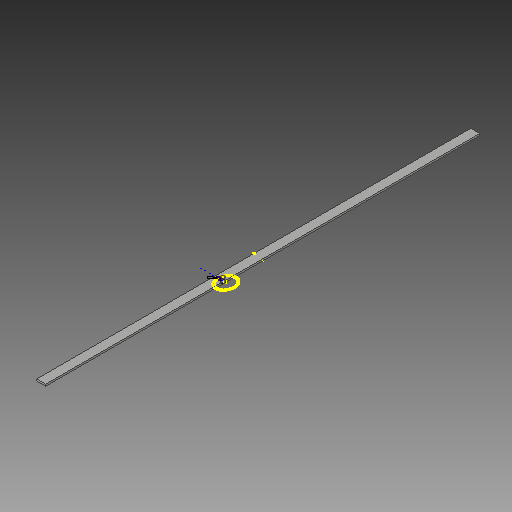
# Autodesk Inventor part: håndfang
Saved by Autodesk Inventor 2018 (Build 220112000, 112)
## iProperties
Created: 2019-09-28
Part Number: håndfang
Material: S235JR
Document SubType Name: Modeling
Designer: loppen
Density: 7.85 g/cm^3
Appearance: Light Gray
Mass: 1186.28 g
Surface Area: 727.87 cm^2
Volume: 151.119 cm^3
Author: loppen
Autodesk Inventor part; units mm, degrees
ref_plane "YZ Plane" through (0, 0, 0) normal (1, 0, 0) x (0, 1, 0)
ref_plane "XZ Plane" through (0, 0, 0) normal (0, 1, 0) x (-1, 0, 0)
ref_plane "XY Plane" through (0, 0, 0) normal (0, 0, 1) x (1, 0, 0)
sketch "Sketch1" plane through (0, 0, 0) normal (0, 0, 1) x (1, 0, 0)
  line L0 (0, 0) -> (25, 0)
  line L1 (25, 0) -> (25, 5)
  line L2 (25, 5) -> (0, 5)
  line L3 (0, 5) -> (0, 0)
  dimension "d0" = 25
  dimension "d1" = 5
  constraints: 8 end point, 2 parallel, 1 horizontal, 1 perpendicular
  measures "d0" distance of L0.start L0.end
  measures "d1" distance of L0.end L1.end
extrude "Extrusion1" add sketch "Sketch1" along normal mid plane 1208.95
sketch "Sketch2" plane through (0, 5, 604.475) normal (0, 1, 0) x (1, 0, 0)
  ellipse E0 centre (30, 495.5291) end of major axis (30, 524.884) minor radius 24.25 projected
  ellipse E1 centre (30, 495.5291) end of major axis (30, 520.3446) minor radius 20.5 projected
  line L0 (30, 495.5291) -> (-41.6864, 495.5291) construction
  circle A0 centre (9.75, 495.5291) radius 4
  line L1 (5.75, 490.0205) -> (5.75, 504.8996) construction
  point P0 (0, 604.475)
  dimension "d4" = 8
  constraints: 4 end point, 1 centre point, 1 horizontal, 1 perpendicular, 1 point on line, 1 tangent, 1 vertical, 2 other
  measures "d4" diameter of A0
body "Solid1"
